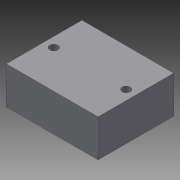
# Autodesk Inventor part: Big_Easy_Stepper_Driver
Saved by Autodesk Inventor 2015 (Build 190159000, 159)
## iProperties
Created: 2015-01-04
Part Number: Big_Easy_Stepper_Driver
Material: Generic
Document SubType Name: Modeling
Designer: ericd_000
Density: 1 g/cm^3
Appearance: Default
Author: ericd_000
Autodesk Inventor part; units mm, degrees
ref_plane "YZ Plane" through (0, 0, 0) normal (1, 0, 0) x (0, 1, 0)
ref_plane "XZ Plane" through (0, 0, 0) normal (0, 1, 0) x (-1, 0, 0)
ref_plane "XY Plane" through (0, 0, 0) normal (0, 0, 1) x (1, 0, 0)
sketch "Sketch1" plane through (0, 0, 0) normal (0, 0, 1) x (1, 0, 0)
  line L0 (-18.5, 15.25) -> (18.5, 15.25)
  line L1 (18.5, 15.25) -> (18.5, -15.25)
  line L2 (18.5, -15.25) -> (-18.5, -15.25)
  line L3 (-18.5, -15.25) -> (-18.5, 15.25)
  point P0 (0, 0)
  point P1 (0, 15.25)
  point P2 (18.5, 0)
  dimension "d0" = 37
  dimension "d1" = 30.5
  constraints: 8 end point, 2 midpoint, 2 parallel, 1 horizontal, 1 horizontal alignment, 1 perpendicular, 1 vertical alignment
  measures "d0" distance of L1.end L2.end
  measures "d1" distance of L0.end L1.end
extrude "Extrusion1" add sketch "Sketch1" along normal blind 15
sketch "Sketch2" plane through (0, 0, 15) normal (0, 0, 1) x (1, 0, 0)
  circle A0 centre (14.605, 0) radius 1.65
  circle A1 centre (-14.605, 0) radius 1.65
  line L0 (14.605, 0) -> (-14.605, 0) construction
  point P0 (0, 0)
  point P1 (0, 0)
  dimension "d4" = 3.3
  dimension "d5" = 3.3
  dimension "d6" = 29.21
  constraints: 2 centre point, 2 end point, 2 horizontal alignment, 1 coincident, 1 horizontal, 1 midpoint
  measures "d4" diameter of A0
  measures "d5" diameter of A1
  measures "d6" distance of L0.start L0.end
extrude "Extrusion2" cut sketch "Sketch2" against normal up to next
body "Solid1"
